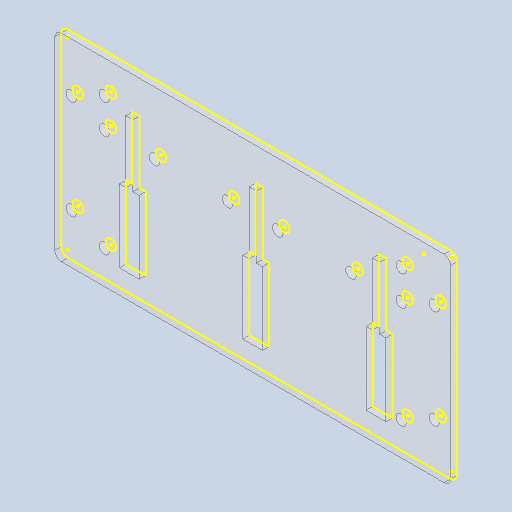
# Autodesk Inventor part: part1
Saved by Autodesk Inventor 2025.2 (Build 292293000, 293)
## iProperties
Created: 2025-02-28
Part Number: part1
Material: アクリル、クリア
Document SubType Name: Modeling
Designer: haruy
Density: 1.19 g/cm^3
Appearance: 透明 - クリア
Author: haruy
Autodesk Inventor part; units mm, degrees
ref_plane "YZ Plane" through (0, 0, 0) normal (1, 0, 0) x (0, 1, 0)
ref_plane "XZ Plane" through (0, 0, 0) normal (0, 1, 0) x (-1, 0, 0)
ref_plane "XY Plane" through (0, 0, 0) normal (0, 0, 1) x (1, 0, 0)
derived "oikon-Sketch-Base.ipt"
sketch "スケッチ1" plane through (100, 0, 0) normal (1, 0, 0) x (0, 1, 0)
  line L0 (0, 0) -> (-50, 0)
  line L1 (-50, 0) -> (-50, -2)
  line L2 (-50, -2) -> (0, -2)
  line L3 (0, -2) -> (0, 0)
  circle A0 centre (-10, -6) radius 4
  circle A1 centre (-10, -6) radius 7
  line L4 (-26, 13) -> (-45, 13)
  line L5 (-45, 13) -> (-45, 2.35)
  line L6 (-45, 2.35) -> (-26, 2.35)
  line L7 (-26, 2.35) -> (-26, 13)
  line L8 (0, 14.6) -> (-50, 14.6)
  line L9 (-50, 14.6) -> (-50, 13)
  line L10 (-50, 13) -> (0, 13)
  line L11 (0, 13) -> (0, 14.6)
  line L12 (0, 36.6) -> (-50, 36.6)
  line L13 (-50, 36.6) -> (-50, 34.6)
  line L14 (-50, 34.6) -> (0, 34.6)
  line L15 (0, 34.6) -> (0, 36.6)
  line L16 (-12.427, 0.5658) -> (-40.5661, -9.8358)
  arc A2 (-34, 2.35) -> (-32, 2.35) centre (-33, 2.35) ccw
  line L17 (-7.573, -12.5658) -> (-35.712, -22.9674)
  line L18 (-40.5661, -9.8358) -> (-35.712, -22.9674)
  line L19 (-35.712, -22.9674) -> (-28.7776, -41.7268)
  arc A3 (-35.712, -22.9674) -> (-32.2448, -32.3471) centre (-33.9784, -27.6572) ccw
  line L20 (-32.2448, -32.3471) -> (-27.555, -30.6135)
  line L21 (-27.555, -30.6135) -> (-26.1339, -34.4579)
  arc A4 (-24.0878, -39.9932) -> (-27.555, -30.6135) centre (-25.8214, -35.3033) ccw
  line L22 (-24.0878, -39.9932) -> (-28.7776, -41.7268)
  arc A5 (-40.5661, -9.8358) -> (-28.7776, -41.7268) centre (-34.6719, -25.7813) ccw
  line L23 (0, 0) -> (5, 0)
  line L24 (5, 0) -> (5, -2)
  line L25 (5, -2) -> (0, -2)
  line L26 (0, -2) -> (0, 0)
  line L27 (0, 36.6) -> (5, 36.6)
  line L28 (5, 36.6) -> (5, 34.6)
  line L29 (5, 34.6) -> (0, 34.6)
  line L30 (0, 34.6) -> (0, 36.6)
  line L31 (-50, 36.6) -> (-55, 36.6)
  line L32 (-55, 36.6) -> (-55, 34.6)
  line L33 (-55, 34.6) -> (-50, 34.6)
  line L34 (-50, 34.6) -> (-50, 36.6)
  line L35 (-50, 0) -> (-55, 0)
  line L36 (-55, 0) -> (-55, -2)
  line L37 (-55, -2) -> (-50, -2)
  line L38 (-50, -2) -> (-50, 0)
  arc A6 (-26.4966, -4.635) -> (-40.5661, -9.8358) centre (-33.5313, -7.2354) ccw
  point P0 (-14.1989, 2.35)
sketch "スケッチ2" plane through (0, 0, 0) normal (0, 0, 1) x (1, 0, 0)
  line L0 (0, 0) -> (-100, 0)
  line L1 (-100, 0) -> (-100, -50)
  line L2 (-100, -50) -> (0, -50)
  line L3 (0, -50) -> (0, 0)
  line L4 (0, -9) -> (-25.2, -9)
  line L5 (-25.2, -9) -> (-25.2, -17)
  line L6 (-25.2, -17) -> (0, -17)
  line L7 (0, -17) -> (0, -9)
  line L8 (0, -50) -> (10, -50)
  line L9 (10, -50) -> (10, 0)
  line L10 (10, 0) -> (0, 0)
  line L11 (0, 0) -> (0, -50)
  line L12 (-100, -50) -> (-110, -50)
  line L13 (-110, -50) -> (-110, 0)
  line L14 (-110, 0) -> (-100, 0)
  line L15 (-100, 0) -> (-100, -50)
  line L16 (-10.1, -7) -> (-15.1, -7)
  line L17 (-15.1, -7) -> (-15.1, -25.7)
  line L18 (-15.1, -25.7) -> (-10.1, -25.7)
  line L19 (-10.1, -25.7) -> (-10.1, -7)
  circle A0 centre (-5, -14) radius 1.6
  line L20 (-12.6, -25.7) -> (-12.6, -7)
  circle A1 centre (-20.2, -14) radius 1.6
  line L21 (-37.4, -9) -> (-62.6, -9)
  line L22 (-62.6, -9) -> (-62.6, -17)
  line L23 (-62.6, -17) -> (-37.4, -17)
  line L24 (-37.4, -17) -> (-37.4, -9)
  circle A2 centre (-42.4, -14) radius 1.6
  circle A3 centre (-57.6, -14) radius 1.6
  circle A4 centre (-79.8, -14) radius 1.6
  circle A5 centre (-95, -14) radius 1.6
  circle A6 centre (5, -10) radius 1.6
  circle A7 centre (5, -40) radius 1.6
  line L25 (-50, 0) -> (-50, -50)
  circle A8 centre (-105, -10) radius 1.6
  circle A9 centre (-105, -40) radius 1.6
  line L26 (-47.5, -6) -> (-52.5, -6)
  line L27 (-52.5, -6) -> (-52.5, -47.8)
  line L28 (-52.5, -47.8) -> (-47.5, -47.8)
  line L29 (-47.5, -47.8) -> (-47.5, -6)
  line L30 (-84.9, -7) -> (-89.9, -7)
  line L31 (-89.9, -7) -> (-89.9, -36.3712)
  line L32 (-89.9, -36.3712) -> (-84.9, -36.3712)
  line L33 (-84.9, -36.3712) -> (-84.9, -7)
  line L34 (10, 0) -> (-110, 0)
  line L35 (-110, 0) -> (-110, 5)
  line L36 (-110, 5) -> (10, 5)
  line L37 (10, 5) -> (10, 0)
  line L38 (10, -50) -> (-110, -50)
  line L39 (-110, -50) -> (-110, -55)
  line L40 (-110, -55) -> (10, -55)
  line L41 (10, -55) -> (10, -50)
  circle A10 centre (-5, -5) radius 1.6
  line L42 (10, -25) -> (-100, -25)
  circle A11 centre (-5, -45) radius 1.6
  circle A12 centre (-95, -45) radius 1.6
  circle A13 centre (-95, -5) radius 1.6
  line L43 (-15.2, -6.9) -> (-10, -6.9)
  line L44 (-10, -6.9) -> (-10, -25.8)
  line L45 (-10, -25.8) -> (-15.2, -25.8)
  line L46 (-15.2, -25.8) -> (-15.2, -6.9)
  line L47 (-9.6, -47.8) -> (-15.6, -47.8)
  line L48 (-15.6, -47.8) -> (-15.6, -25.8)
  line L49 (-15.6, -25.8) -> (-9.6, -25.8)
  line L50 (-9.6, -25.8) -> (-9.6, -47.8)
  line L51 (-53, -47.8) -> (-53, -25.8)
  line L52 (-47, -47.8) -> (-53, -47.8)
  line L53 (-47, -25.8) -> (-47, -47.8)
  line L54 (-53, -25.8) -> (-47, -25.8)
  line L55 (-47.4, -6.9) -> (-47.4, -25.8)
  line L56 (-52.6, -25.8) -> (-52.6, -6.9)
  line L57 (-52.6, -6.9) -> (-47.4, -6.9)
  line L58 (-90.4, -47.8) -> (-90.4, -25.8)
  line L59 (-84.4, -47.8) -> (-90.4, -47.8)
  line L60 (-84.4, -25.8) -> (-84.4, -47.8)
  line L61 (-90.4, -25.8) -> (-84.4, -25.8)
  line L62 (-84.8, -6.9) -> (-84.8, -25.8)
  line L63 (-90, -25.8) -> (-90, -6.9)
  line L64 (-90, -6.9) -> (-84.8, -6.9)
  line L65 (-11.6, -25.8) -> (-13.6, -25.8)
  line L66 (-13.6, -25.8) -> (-13.6, -6.9)
  line L67 (-13.6, -6.9) -> (-11.6, -6.9)
  line L68 (-11.6, -6.9) -> (-11.6, -25.8)
  line L69 (-11.5, -25.9) -> (-13.7, -25.9)
  line L70 (-13.7, -25.9) -> (-13.7, -6.8)
  line L71 (-13.7, -6.8) -> (-11.5, -6.8)
  line L72 (-11.5, -6.8) -> (-11.5, -25.9)
  line L73 (-48.9, -25.9) -> (-51.1, -25.9)
  line L74 (-48.9, -6.8) -> (-48.9, -25.9)
  line L75 (-51.1, -25.9) -> (-51.1, -6.8)
  line L76 (-51, -25.8) -> (-51, -6.9)
  line L77 (-49, -6.9) -> (-49, -25.8)
  line L78 (-51.1, -6.8) -> (-48.9, -6.8)
  line L79 (-86.3, -25.9) -> (-88.5, -25.9)
  line L80 (-86.3, -6.8) -> (-86.3, -25.9)
  line L81 (-88.5, -25.9) -> (-88.5, -6.8)
  line L82 (-88.4, -25.8) -> (-88.4, -6.9)
  line L83 (-86.4, -6.9) -> (-86.4, -25.8)
  line L84 (-88.5, -6.8) -> (-86.3, -6.8)
  point P0 (-52.6, -25.8)
  point P1 (-47.4, -25.8)
  point P2 (-10, -25.8)
  point P3 (-15.2, -25.8)
  point P4 (-90, -25.8)
  point P5 (-84.8, -25.8)
  point P6 (-88.5, -6.9)
  point P7 (-88.5, -25.8)
  point P8 (-86.3, -6.9)
  point P9 (-86.3, -25.8)
  point P10 (-51.1, -6.9)
  point P11 (-51.1, -25.8)
  point P12 (-48.9, -6.9)
  point P13 (-48.9, -25.8)
  point P14 (-13.7, -6.9)
  point P15 (-13.7, -25.8)
  point P16 (-11.5, -6.9)
  point P17 (-11.5, -25.8)
ref_plane "作業平面1" through (100, 0, 0) normal (1, 0, 0) x (0, 1, 0)
extrude "押し出し1" add sketch "スケッチ2" along normal blind 2 contours L3 L4 L44 L43 L72 L71 L70 L46 L5 L6 L42 L55 L23 L24 L21 L57 L29 L26 L25 L0 | L10 L9 L42 L3 | L0 L14 L35 L36 L37 L10 | L25 L26 L27 L57 L56 L21 L22 L23 L42 L62 L64 L80 L84 L81 L63 L1 L0 | L3 L6 L44 L4 | L1 L12 L13 L14 | L26 L29 L57 L74 L78 L25 | L25 L78 L75 L57 L27 L26 | L3 L42 L44 L6 | L9 L8 L3 L42 | L42 L63 L61 L58 L59 L60 L62 L56 L54 L51 L52 L28 L25 L2 L1 | L78 L74 L57 L25 | L25 L57 L75 L78 | L3 L2 L25 L28 L52 L53 L54 L55 L42 L46 L49 L48 L47 L50 L44 | L41 L40 L39 L12 L2 L8 | L43 L70 L71 L72 | L81 L84 L80 L64 | L21 L24 L23 L55 | L56 L23 L22 L21 | L46 L6 L5 L4
fillet "フィレット1" radius 2 4 edges at (10, 5, 1) (10, -55, 1) (-110, -55, 1) (-110, 5, 1)
extrude "押し出し2" add sketch "スケッチ2" along normal blind 2 contours L44 L6 L19 L4 | L4 L19 L16 L72 L43 L44 | L44 L42 L19 L6 | L19 L6 L72 L4 | L4 L72 L16 L19 | L63 L64 L81 L30 L31 L42 | L42 L31 L61 L63 | L57 L55 L21 L29 | L29 L21 L74 L57 | L57 L75 L21 L27 | L27 L21 L56 L57 | L44 L45 L72 L18 L19 L42 | L19 L42 L72 L6 | L42 L81 L61 L31 | L31 L30 L81 L42 | L29 L23 L74 L21 | L21 L55 L23 L29 | L27 L23 L56 L21 | L21 L75 L23 L27 | L19 L18 L72 L42 | L29 L42 L74 L23 | L23 L55 L42 L29 | L27 L42 L56 L23 | L23 L75 L42 L27 | L42 L55 L54 L29 | L29 L54 L74 L42 | L42 L75 L54 L27 | L27 L54 L56 L42 | L70 L16 L17 L4 L46 L43 | L70 L6 L17 L4 | L4 L17 L16 L70 | L61 L80 L42 L33 | L33 L42 L62 L61 | L80 L30 L33 L42 | L64 L62 L42 L33 L30 L80 | L46 L6 L17 L42 | L42 L17 L18 L70 L45 L46 | L70 L42 L17 L6 | L17 L6 L46 L4 | L42 L70 L18 L17
sketch "スケッチ3" plane through (8, 5, 0) normal (0, 0, -1) x (-1, 0, 0)
  arc A0 (118, -2) -> (116, 0) centre (116, -2) ccw projected
  line L0 (0, 0) -> (116, 0) projected
  arc A1 (0, 0) -> (-2, -2) centre (0, -2) ccw projected
  line L1 (-2, -58) -> (-2, -2) projected
  arc A2 (-2, -58) -> (0, -60) centre (0, -58) ccw projected
  line L2 (116, -60) -> (0, -60) projected
  arc A3 (116, -60) -> (118, -58) centre (116, -58) ccw projected
  line L3 (118, -2) -> (118, -58) projected
  circle A4 centre (65.6, -19) radius 1.6 projected
  line L4 (61, -52.8) -> (61, -30.8) projected
  line L5 (55, -52.8) -> (61, -52.8) projected
  line L6 (55, -30.8) -> (55, -52.8) projected
  line L7 (56.9, -30.8) -> (55, -30.8) projected
  line L8 (56.9, -11.9) -> (56.9, -30.8) projected
  line L9 (59.1, -11.9) -> (56.9, -11.9) projected
  line L10 (59.1, -30.8) -> (59.1, -11.9) projected
  line L11 (61, -30.8) -> (59.1, -30.8) projected
  line L12 (19.5, -30.8) -> (17.6, -30.8) projected
  line L13 (19.5, -11.9) -> (19.5, -30.8) projected
  line L14 (21.7, -11.9) -> (19.5, -11.9) projected
  line L15 (21.7, -30.8) -> (21.7, -11.9) projected
  line L16 (23.6, -30.8) -> (21.7, -30.8) projected
  line L17 (23.6, -52.8) -> (23.6, -30.8) projected
  line L18 (17.6, -52.8) -> (23.6, -52.8) projected
  line L19 (17.6, -30.8) -> (17.6, -52.8) projected
  circle A5 centre (13, -19) radius 1.6 projected
  circle A6 centre (28.2, -19) radius 1.6 projected
  circle A7 centre (50.4, -19) radius 1.6 projected
  circle A8 centre (3, -15) radius 1.6 projected
  circle A9 centre (13, -10) radius 1.6 projected
  circle A10 centre (13, -50) radius 1.6 projected
  circle A11 centre (3, -45) radius 1.6 projected
  circle A12 centre (113, -45) radius 1.6 projected
  circle A13 centre (113, -15) radius 1.6 projected
  circle A14 centre (103, -50) radius 1.6 projected
  circle A15 centre (87.8, -19) radius 1.6 projected
  circle A16 centre (103, -19) radius 1.6 projected
  circle A17 centre (103, -10) radius 1.6 projected
  line L20 (92.4, -30.8) -> (92.4, -52.8) projected
  line L21 (94.3, -30.8) -> (92.4, -30.8) projected
  line L22 (94.3, -11.9) -> (94.3, -30.8) projected
  line L23 (96.5, -11.9) -> (94.3, -11.9) projected
  line L24 (96.5, -30.8) -> (96.5, -11.9) projected
  line L25 (98.4, -30.8) -> (96.5, -30.8) projected
  line L26 (98.4, -52.8) -> (98.4, -30.8) projected
  line L27 (92.4, -52.8) -> (98.4, -52.8) projected
  point P0 (8, -5)
